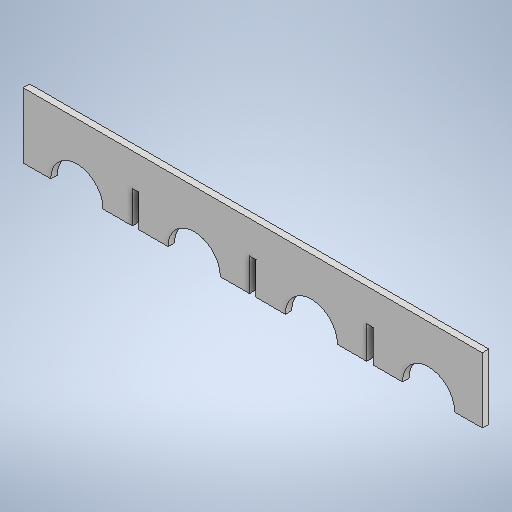
# Autodesk Inventor part: BSH 086 amplifier bottom
Saved by Autodesk Inventor 2025 (Build 290162010, 162A)
## iProperties
Created: 2024-08-04
Part Number: BSH 086 amplifier bottom
Material: Stainless Steel
Document SubType Name: Sheet Metal
Designer: pokla
Density: 8 g/cm^3
Sheet Metal Rule: AISI304 2mm Die16
Appearance: Default
Author: pokla
Autodesk Inventor part; units mm, degrees
ref_plane "YZ Plane" through (0, 0, 0) normal (1, 0, 0) x (0, 1, 0)
ref_plane "XZ Plane" through (0, 0, 0) normal (0, 1, 0) x (-1, 0, 0)
ref_plane "XY Plane" through (0, 0, 0) normal (0, 0, 1) x (1, 0, 0)
sketch "Sketch1" plane through (0, 0, 0) normal (0, 0, 1) x (1, 0, 0)
  circle A0 centre (0, 0) radius 400 construction
  line L0 (-352.5, 175) -> (352.5, 175)
  line L1 (352.5, 175) -> (352.5, 185)
  line L2 (352.5, 185) -> (-352.5, 185)
  line L3 (-352.5, 185) -> (-352.5, 175)
  line L4 (-352.5, 175) -> (352.5, 185) construction
  point P0 (0, 180)
  dimension "d0" = 800
  dimension "d32" = 10
  dimension "d33" = 180
  dimension "d34" = 705
  constraints: 10 end point, 3 coincident, 2 parallel, 1 centre point, 1 horizontal, 1 midpoint, 1 perpendicular, 1 vertical alignment
  measures "d0" diameter of A0
  measures "d32" distance between parallel lines of L0 L2
  measures "d33" distance of point (0, 0) point (0, 180)
  measures "d34" distance of L1.end L2.end
extrude "Extrusion1" add sketch "Sketch1" along normal blind 100
sketch "Sketch3" plane through (-352.5, 175, 0) normal (0, -1, 0) x (1, 0, 0)
  line L0 (705, 0) -> (0, 0) projected
  circle A0 centre (262.5, 0) radius 40
  circle A1 centre (82.5, 0) radius 40
  circle A2 centre (442.5, 0) radius 40
  circle A3 centre (622.5, 0) radius 40
  line L1 (0, 0) -> (705, 0) projected
  line L2 (0, 100) -> (705, 100) projected
  line L3 (167.5, 50) -> (177.5, 50)
  line L4 (177.5, 50) -> (177.5, 0)
  line L5 (177.5, 0) -> (167.5, 0)
  line L6 (167.5, 0) -> (167.5, 50)
  line L7 (347.5, 50) -> (357.5, 50)
  line L8 (357.5, 50) -> (357.5, 0)
  line L9 (357.5, 0) -> (347.5, 0)
  line L10 (347.5, 0) -> (347.5, 50)
  line L11 (527.5, 50) -> (537.5, 50)
  line L12 (537.5, 50) -> (537.5, 0)
  line L13 (537.5, 0) -> (527.5, 0)
  line L14 (527.5, 0) -> (527.5, 50)
  point P0 (352.5, 0)
  point P1 (352.5, 0)
  point P2 (352.5, 0)
  point P3 (582.5, 0)
  point P4 (662.5, 0)
  point P5 (402.5, 0)
  point P6 (482.5, 0)
  point P7 (222.5, 0)
  point P8 (302.5, 0)
  point P9 (42.5, 0)
  point P10 (122.5, 0)
  point P11 (172.5, 0)
  point P12 (352.5, 0)
  point P13 (352.5, 0)
  point P14 (352.5, 0)
  point P15 (532.5, 0)
  point P16 (352.5, 0)
  point P17 (352.5, 0)
  point P18 (527.5, 0)
  point P19 (537.5, 0)
  point P20 (357.5, 0)
  point P21 (177.5, 0)
  dimension "d35" = 80
  dimension "d36" = 90
  dimension "d37" = 80
  dimension "d38" = 180
  dimension "d39" = 80
  dimension "d40" = 80
  dimension "d41" = 90
  dimension "d42" = 180
  dimension "d53" = 10
  dimension "d54" = 180
  dimension "d55" = 50
  dimension "d56" = 10
  dimension "d57" = 50
  dimension "d58" = 10
  dimension "d59" = 50
  dimension "d60" = 180
  constraints: 24 end point, 6 parallel, 4 centre point, 3 horizontal, 3 midpoint, 3 perpendicular, 2 horizontal alignment, 13 other
  measures "d35" diameter of A0
  measures "d36" distance of point (352.5, 0) A0.centre
  measures "d37" diameter of A1
  measures "d38" distance of A0.centre A1.centre
  measures "d39" diameter of A2
  measures "d40" diameter of A3
  measures "d41" distance of point (352.5, 0) A2.centre
  measures "d42" distance of A2.centre A3.centre
  measures "d53" distance between parallel lines of L6 L4
  measures "d54" distance of point (352.5, 0) point (172.5, 0)
  measures "d55" distance of L5.end L3.start
  measures "d56" distance between parallel lines of L10 L8
  measures "d57" distance of L9.end L7.start
  measures "d58" distance between parallel lines of L14 L12
  measures "d59" distance of L13.end L11.start
  measures "d60" distance of point (532.5, 0) point (352.5, 0)
extrude "Extrusion3" cut sketch "Sketch3" against normal through all contours L0 A1 | L0 L6 L3 L4 | L0 A0 | L0 L10 L7 L8 | L0 A2 | A3 L0 | L0 L14 L11 L12 picked at (84.0738, 20.5179) picked at (255.8333, 20.5179) picked at (435.8333, 20.5179) picked at (611.7131, 7.8371)
equation "\"d56\" = d53"
equation "\"d57\" = d55"
equation "\"d58\" = d56"
equation "\"d59\" = d57"
equation "\"d60\" = d54"
equation "\"BendReliefWidth\" = Thickness"
equation "\"BendReliefDepth\" = 0.5 * Thickness"
equation "\"CornerReliefSize\" = 4 * Thickness"
equation "\"MinimumRemnant\" = 2 * Thickness"
equation "\"TransitionRadius\" = BendRadius"
equation "\"JacobiRadiusSize\" = BendRadius"
equation "\"GapSize\" = Thickness"
equation "\"Thickness\" = 2"
equation "\"BendRadius\" = 2.75"
body "Solid1"
